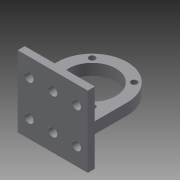
# Autodesk Inventor part: ff12_mount
Saved by Autodesk Inventor 2014 (Build 180170000, 170)
## iProperties
Created: 2014-08-22
Part Number: ff12_mount
Material: Generic
Document SubType Name: Modeling
Designer: Matthew
Density: 1 g/cm^3
Appearance: Default
Mass: 21.0838 g
Surface Area: 105.452 cm^2
Volume: 21.0838 cm^3
Author: Matthew
Autodesk Inventor part; units mm, degrees
ref_plane "YZ Plane" through (0, 0, 0) normal (1, 0, 0) x (0, 1, 0)
ref_plane "XZ Plane" through (0, 0, 0) normal (0, 1, 0) x (-1, 0, 0)
ref_plane "XY Plane" through (0, 0, 0) normal (0, 0, 1) x (1, 0, 0)
sketch "Sketch1" plane through (0, 0, 0) normal (0, 0, 1) x (1, 0, 0)
  circle A0 centre (0, 0) radius 17
  arc A1 (25, 0) -> (-25, 0) centre (0, 0) ccw
  line L0 (-25, 0) -> (-25, -23.1305)
  line L1 (-25, -23.1305) -> (25, -23.1305)
  line L2 (25, -23.1305) -> (25, 0)
  circle A2 centre (-15, 15) radius 2.25
  circle A3 centre (15, 15) radius 2.25
  circle A4 centre (-15, -15) radius 2.25
  circle A5 centre (15, -15) radius 2.25
  dimension "d0" = 34
  dimension "d1" = 50
  dimension "d2" = 50
  dimension "d3" = 23.1305
  dimension "d54" = 4.5
  dimension "d57" = 30
  dimension "d60" = 30
  dimension "d63" = 15
  dimension "d64" = 15
  constraints: 6 centre point, 6 end point, 2 coincident, 2 point on circle, 2 tangent, 2 vertical, 1 horizontal, 1 perpendicular, 6 other
  measures "d0" diameter of A0
  measures "d1" diameter of A1
  measures "d2" distance of L0.end L1.end
  measures "d3" distance of L1.end L2.end
  measures "d54" diameter of A2
  measures "d57" distance of A2.centre A3.centre
  measures "d60" distance of A2.centre A4.centre
  measures "d63" horizontal distance of point (0, 0) A4.centre
  measures "d64" horizontal distance of A2.centre point (0, 0)
extrude "Extrusion1" add sketch "Sketch1" along normal blind 8 contours L2 L1 L0 A1 | A2 | A3 | A4 | A5
sketch "Sketch2" plane through (-25, -23.1305, 0) normal (0, -1, 0) x (1, 0, 0)
  line L0 (0, 0) -> (50, 0) construction
  line L1 (0, 0) -> (0, 8) projected
  line L2 (0, -21.4) -> (50, -21.4)
  line L3 (50, -21.4) -> (50, 29.4)
  line L4 (50, 29.4) -> (0, 29.4)
  line L5 (0, 29.4) -> (0, -21.4)
  line L6 (0, -21.4) -> (50, 29.4) construction
  line L7 (50, -21.4) -> (0, 29.4) construction
  point P0 (25, 0)
  point P1 (25, 4)
  point P2 (25, 4)
  point P3 (0, 4)
  point P4 (25, 4)
  point P5 (25, 0)
  point P6 (50, 8)
  dimension "d7" = 50.8
  dimension "d65" = 50
  dimension "d66" = 50
  constraints: 12 end point, 6 midpoint, 2 parallel, 1 horizontal, 1 horizontal alignment, 1 perpendicular, 1 vertical alignment
  measures "d7" distance of L2.end L3.end
  measures "d65" distance of L3.end L4.end
  measures "d66" distance of L1.end point (50, 8)
extrude "Extrusion2" add sketch "Sketch2" along normal blind 5
sketch "Sketch3" plane through (-25, -28.1305, 0) normal (0, -1, 0) x (1, 0, 0)
  line L0 (50, 29.4) -> (0, 29.4) projected
  line L1 (0, 29.4) -> (0, -21.4) projected
  point P0 (25, 0)
  point P1 (8.0667, 16.7)
  point P2 (25, 16.7)
  point P3 (8.0667, -8.7)
  point P4 (25, -8.7)
  point P5 (41.9333, 16.7)
  point P6 (41.9333, -8.7)
  dimension "d39" = 16.9333
  dimension "d42" = 25.4
  dimension "d45" = 12.7
  dimension "d67" = 50
  dimension "d68" = 50.8
  dimension "d70" = 8.0667
  constraints: 1 horizontal, 1 vertical, 5 other
  measures "d39" distance of point (8.067, 16.7) point (25, 16.7)
  measures "d42" distance of point (8.067, 16.7) point (8.067, -8.7)
  measures "d45" distance from line of L0 point (8.067, 16.7)
  measures "d67" distance of L0.start L0.end
  measures "d68" distance of L0.end L1.end
  measures "d70" distance from line of L1 point (8.067, 16.7)
hole "Hole2" at (-16.9333, -28.1305, 16.7) at (0, -28.1305, 16.7) at (-16.9333, -28.1305, -8.7) at (0, -28.1305, -8.7) at (16.9333, -28.1305, 16.7) at (16.9333, -28.1305, -8.7) direction (0, 1, 0) diameter 6.35 end through all
sketch "Sketch4" plane through (0, 0, 0) normal (0, 0, -1) x (-1, 0, 0)
  circle A0 centre (0, 0) radius 17 projected
  line L0 (25, 0) -> (25, -23.1305) projected
  line L1 (25, -23.1305) -> (-25, -23.1305) projected
  point P0 (-15, 15)
  point P1 (15, 15)
  point P2 (-15, -15)
  point P3 (15, -15)
  dimension "d80" = 30
  dimension "d83" = 30
  dimension "d86" = 15
  dimension "d87" = 15
  constraints: 1 horizontal, 1 vertical, 3 other
  measures "d80" distance of point (-15, 15) point (15, 15)
  measures "d83" distance of point (-15, 15) point (-15, -15)
  measures "d86" horizontal distance of A0.centre point (-15, 15)
  measures "d87" horizontal distance of point (-15, 15) A0.centre
hole "Hole3" at (15, 15, 0) at (-15, 15, 0) at (15, -15, 0) at (-15, -15, 0) direction (0, 0, 1) diameter 4.5 end through all
equation "\"d2\" = d1"
equation "\"d63\" = 0.5 * d60"
equation "\"d64\" = d63"
equation "\"d65\" = d66"
equation "\"d70\" = -d39 + 0.5 * d67"
equation "\"d83\" = d80"
equation "\"d86\" = 0.5 * d80"
equation "\"d87\" = d86"
body "Solid1"
